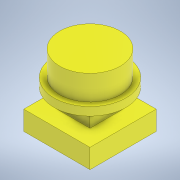
# Autodesk Inventor part: Bouton
Saved by Autodesk Inventor 2020 (Build 240168000, 168)
## iProperties
Created: 2020-01-01
Part Number: Bouton
Material: Argent
Document SubType Name: Modeling
Designer: Manuel Enzo
Density: 10.49 g/cm^3
Appearance: Jaune
Author: Manuel Enzo
Autodesk Inventor part; units mm, degrees
ref_plane "YZ Plane" through (0, 0, 0) normal (1, 0, 0) x (0, 1, 0)
ref_plane "XZ Plane" through (0, 0, 0) normal (0, 1, 0) x (-1, 0, 0)
ref_plane "XY Plane" through (0, 0, 0) normal (0, 0, 1) x (1, 0, 0)
sketch "Esquisse1" plane through (0, 0, 0) normal (0, 1, 0) x (-1, 0, 0)
  line L0 (0, 0) -> (12, 0)
  line L1 (12, 0) -> (12, -12)
  line L2 (12, -12) -> (0, -12)
  line L3 (0, -12) -> (0, 0)
  dimension "d0" = 12
  dimension "d1" = 12
  constraints: 8 end point, 2 parallel, 1 horizontal, 1 perpendicular
  measures "d0" distance between parallel lines of L3 L1
  measures "d1" distance between parallel lines of L0 L2
extrude "Extrusion1" add sketch "Esquisse1" along normal blind 3.5
sketch "Esquisse2" plane through (0, 3.5, 0) normal (0, 1, 0) x (1, 0, 0)
  line L0 (-9, 3) -> (-3, 3)
  line L1 (-3, 3) -> (-3, 9)
  line L2 (-3, 9) -> (-9, 9)
  line L3 (-9, 9) -> (-9, 3)
  line L4 (0, 0) -> (0, 12) projected
  line L5 (-12, 12) -> (-12, 0) projected
  line L6 (-12, 0) -> (0, 0) projected
  dimension "d4" = 6
  dimension "d5" = 6
  dimension "d6" = 3
  dimension "d7" = 3
  dimension "d8" = 3
  constraints: 8 end point, 2 parallel, 1 horizontal, 1 perpendicular
  measures "d4" distance between parallel lines of L0 L2
  measures "d5" distance between parallel lines of L3 L1
  measures "d6" distance between parallel lines of L4 L1
  measures "d7" distance between parallel lines of L5 L3
  measures "d8" distance between parallel lines of L6 L0
extrude "Extrusion2" add sketch "Esquisse2" along normal blind 3.5
sketch "Esquisse3" plane through (0, 7, 0) normal (0, 1, 0) x (1, 0, 0)
  circle A0 centre (-6, 6) radius 6.5
  circle A1 centre (-6, 6) radius 5.5
  line L0 (-9, 9) -> (-9, 3) projected
  line L1 (-9, 3) -> (-3, 3) projected
  point P0 (0, 0)
  dimension "d11" = 1
  dimension "d12" = 3
  dimension "d13" = 3
  dimension "d14" = 13
  constraints: 2 centre point, 1 coincident
  measures "d11" radial gap between concentric circles of A0 A1
  measures "d12" distance from line of L0 A0.centre
  measures "d13" distance from line of L1 A0.centre
  measures "d14" diameter of A0
extrude "Extrusion3" add sketch "Esquisse3" along normal blind 6 contours A1
extrude "Extrusion4" add sketch "Esquisse3" along normal blind 1.5
